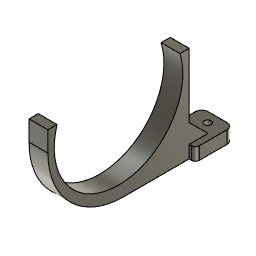
duct-holder (Autodesk Fusion 360 design; units mm, degrees)
Autodesk Fusion 360 part; units mm, degrees
sketch "Sketch1" plane through (0, 0, 0) normal (1, 0, 0) x (0, 1, 0)
  circle A0 centre (0, 0) radius 51
  dimension "d1" = 102
  constraint coincident A0.centre origin
  measures "d1" diameter of A0
extrude "Extrude1" add sketch "Sketch1" along normal blind 32 makes body 1
sketch "Sketch2" plane through (32, 0, 0) normal (1, 0, 0) x (0, 1, 0)
  circle A0 centre (0, 0) radius 51
  circle A1 centre (0, 0) radius 51
  line L0 (-56, 0) -> (56, 0)
  line L1 (56, 0) -> (56, -61)
  line L2 (56, -61) -> (-56, -61)
  line L3 (-56, -61) -> (-56, 0)
  dimension "d5" = 5
  dimension "d6" = 5
  dimension "d7" = 10
  constraint horizontal L0
  constraint vertical L1
  constraint horizontal L2
  constraint vertical L3
  constraint coincident A0.centre L0
  measures "d5" distance of A0 L1
  measures "d6" distance of A0 L3
  measures "d7" distance of A1 L2
extrude "Extrude2" add sketch "Sketch2" against normal blind 15 separate body contours A0 A1 L0 L1 L2 L3 makes body 2
combine "Combine1" operation cut target body 2 tool bodies 1
sketch "Sketch3" plane through (0, 0, 0) normal (0, 0, 1) x (1, 0, 0)
  line L0 (32, -56) -> (17, -56)
  line L1 (32, 56) -> (17, 56)
  line L2 (32, 51) -> (17, 51)
  line L3 (17, 56) -> (17, 51)
  line L4 (32, 51) -> (32, 56)
  line L5 (32, -56) -> (32, -51)
  line L6 (17, -51) -> (17, -56)
  line L7 (32, -51) -> (17, -51)
  line L8 (32, -51) -> (32, 51) construction
  line L9 (17, -51) -> (17, 51) construction
  line L10 (32, 0) -> (0, 0) construction
  line L11 (62, -12.5) -> (32, -12.5)
  line L12 (32, -12.5) -> (32, 12.5)
  line L13 (32, 12.5) -> (62, 12.5)
  line L14 (62, 12.5) -> (62, -12.5)
  line L15 (62, 0) -> (32, 0) construction
  circle A0 centre (54.25, 0) radius 2.75
  circle A1 centre (54.25, 0) radius 1.5
  line L16 (24.5, 56) -> (24.5, 51) construction
  line L17 (37, 56) -> (12, 56)
  line L18 (12, 56) -> (12, 86)
  line L19 (12, 86) -> (37, 86)
  line L20 (37, 86) -> (37, 56)
  line L21 (24.5, 56) -> (24.5, 86) construction
  circle A2 centre (24.5, 78.25) radius 2.75
  circle A3 centre (24.5, 78.25) radius 1.5
  point P0 (32, 56)
  point P1 (54.25, 0)
  dimension "d10" = 30
  dimension "d11" = 25
  dimension "d12" = 5.5
  dimension "d13" = 3
  dimension "d14" = 5
  dimension "d29" = 5.5
  dimension "d30" = 5
  dimension "d31" = 3
  constraint coincident L5.end L7.start
  constraint coincident L2.start L4.start
  constraint coincident L6.start L7.end
  constraint coincident L2.end L3.end
  constraint midpoint L8 L10.start
  constraint coincident L10.end origin
  constraint horizontal L11
  constraint vertical L12
  constraint horizontal L13
  constraint vertical L14
  constraint midpoint L14 L15.start
  constraint midpoint L12 L10.start
  constraint coincident L10.start L15.end
  constraint coincident P1 A0.centre
  constraint concentric A0 A1
  constraint coincident L15 P1
  constraint midpoint L1 L16.start
  constraint midpoint L2 L16.end
  constraint horizontal L17
  constraint vertical L18
  constraint horizontal L19
  constraint vertical L20
  constraint equal L14 L17
  constraint equal L13 L20
  constraint midpoint L17 L16.start
  constraint midpoint L19 L21.end
  constraint coincident L21 A2.centre
  constraint concentric A2 A3
  constraint coincident L16.start L21.start
  measures "d10" distance of L11.start L11.end
  measures "d11" distance of L11.start L13.end
  measures "d12" diameter of A0
  measures "d13" diameter of A1
  measures "d14" distance of L14 A0
  measures "d29" diameter of A2
  measures "d30" distance of L19 A2
  measures "d31" diameter of A3
extrude "Extrude5" add sketch "Sketch3" along normal blind 10 from surface at -61 contours L1 L17 L18 L19 L20 | A2 bodies 2
extrude "Extrude6" cut sketch "Sketch3" against normal blind 5 from surface at -51 contours A2 bodies 2
move_face "OffsetFaces2" offset 15 2 faces at (27, -54.3333, 0) (27, 52.6667, 0) on bodies 2
fillet "Fillet4" radius 5 2 edges at (37, 86, -56) (12, 86, -56) on bodies 2
fillet "Fillet6" radius 60 1 edges at (24.5, -56, -61) on bodies 2
fillet "Fillet7" radius 3 2 edges at (12, 56, -56) (37, 56, -56) on bodies 2
chamfer "Chamfer2" distance 15 angle 45 1 edges at (24.5, 56, -51) on bodies 2
named bodies: "duct-holder"
